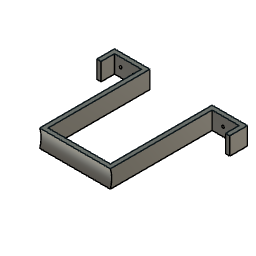
water_level_bracket_v1 (Autodesk Fusion 360 design; units mm, degrees)
Autodesk Fusion 360 part; units mm, degrees
note: some values were not read from the file. Set by a fixed rule: which sketch regions a step uses.
sketch "Sketch1" plane through (0, 0, 0) normal (0, 0, 1) x (1, 0, 0)
  line L0 (0, 0) -> (101.6, 0)
  line L1 (101.6, 0) -> (101.6, 6)
  line L2 (101.6, 6) -> (0, 6)
  line L3 (0, 6) -> (0, 0)
  dimension "d1" = 101.6
  dimension "d2" = 6
  constraint horizontal L0
  constraint vertical L1
  constraint horizontal L2
  constraint vertical L3
  constraint coincident L0.start L3.end
  measures "d1" distance of L0.start L0.end
  measures "d2" distance of L0.end L1.end
extrude "Extrude1" add sketch "Sketch1" along normal blind 25.4
sketch "Sketch2" plane through (0, 0, 25.4) normal (0, 0, 1) x (-1, 0, 0)
  line L0 (0, -6) -> (0, 0)
  line L1 (0, 0) -> (-101.6, 0)
  line L2 (-101.6, 0) -> (-101.6, -6)
  line L3 (-101.6, -6) -> (0, -6)
  line L4 (-101.6, 0) -> (-95.6, 0)
  line L5 (-95.6, 0) -> (-95.6, -152.4)
  line L6 (-95.6, -152.4) -> (-101.6, -152.4)
  line L7 (-101.6, -152.4) -> (-101.6, 0)
  dimension "d5" = 152.4
  dimension "d6" = 6
  constraint horizontal L4
  constraint vertical L5
  constraint horizontal L6
  constraint vertical L7
  constraint coincident L1.end L2.start
  measures "d5" distance of L1.end L6.end
  measures "d6" distance of L5.end L6.end
extrude "Extrude2" add sketch "Sketch2" against normal blind 25.4 contours L3 L5 L6 L7
sketch "Sketch3" plane through (0, 0, 25.4) normal (0, 0, 1) x (-1, 0, 0)
  line L0 (0, -6) -> (0, 0)
  line L1 (0, 0) -> (-101.6, 0)
  line L2 (-101.6, 0) -> (-101.6, -152.4)
  line L3 (-101.6, -152.4) -> (-95.6, -152.4)
  line L4 (-95.6, -152.4) -> (-95.6, -6)
  line L5 (-95.6, -6) -> (0, -6)
  line L6 (0, 0) -> (-6, 0)
  line L7 (-6, 0) -> (-6, -152.4)
  line L8 (-6, -152.4) -> (0, -152.4)
  line L9 (0, -152.4) -> (0, 0)
  dimension "d9" = 152.4
  dimension "d10" = 6
  constraint horizontal L6
  constraint vertical L7
  constraint horizontal L8
  constraint vertical L9
  constraint coincident L0.end L1.start
  measures "d9" distance of L0.end L8.end
  measures "d10" distance of L7.end L8.end
extrude "Extrude3" add sketch "Sketch3" against normal blind 25.4 contours L5 L7 L8 L9
sketch "Sketch4" plane through (101.6, 0, 0) normal (1, 0, 0) x (0, 1, 0)
  line L0 (0, 0) -> (152.4, 0)
  line L1 (152.4, 0) -> (152.4, 25.4)
  line L2 (152.4, 25.4) -> (0, 25.4)
  line L3 (0, 25.4) -> (0, 0)
  circle A0 centre (-39.719, 12.7) radius 41.7
  dimension "d13" = 83.4
  constraint coincident L2.end A0
  constraint coincident L0.start A0
  measures "d13" diameter of A0
extrude "Extrude4" cut sketch "Sketch4" against normal blind 101.6 contours L3 A0 picked at (0.3655, 9.8525)
sketch "Sketch5" plane through (0, 0, 25.4) normal (0, 0, 1) x (-1, 0, 0)
  line L0 (0, -152.4) -> (0, 0)
  line L1 (0, 0) -> (-101.6, 0)
  line L2 (-101.6, 0) -> (-101.6, -152.4)
  line L3 (-101.6, -152.4) -> (-95.6, -152.4)
  line L4 (-95.6, -152.4) -> (-95.6, -6)
  line L5 (-95.6, -6) -> (-6, -6)
  line L6 (-6, -6) -> (-6, -152.4)
  line L7 (-6, -152.4) -> (0, -152.4)
  line L8 (-6, -152.4) -> (44.8, -152.4)
  line L9 (44.8, -152.4) -> (44.8, -146.4)
  line L10 (44.8, -146.4) -> (-6, -146.4)
  line L11 (-6, -146.4) -> (-6, -152.4)
  dimension "d16" = 50.8
  dimension "d17" = 6
  constraint horizontal L8
  constraint vertical L9
  constraint horizontal L10
  constraint vertical L11
  constraint coincident L6.end L7.start
  measures "d16" distance of L6.end L8.end
  measures "d17" distance of L8.end L9.end
extrude "Extrude5" add sketch "Sketch5" against normal blind 25.4 contours L0 L8 L9 L10
sketch "Sketch6" plane through (0, 0, 25.4) normal (0, 0, 1) x (-1, 0, 0)
  line L0 (0, -146.4) -> (0, 0)
  line L1 (0, 0) -> (-101.6, 0)
  line L2 (-101.6, 0) -> (-101.6, -152.4)
  line L3 (-101.6, -152.4) -> (-95.6, -152.4)
  line L4 (-95.6, -152.4) -> (-95.6, -6)
  line L5 (-95.6, -6) -> (-6, -6)
  line L6 (-6, -6) -> (-6, -152.4)
  line L7 (-6, -152.4) -> (44.8, -152.4)
  line L8 (44.8, -152.4) -> (44.8, -146.4)
  line L9 (44.8, -146.4) -> (0, -146.4)
  line L10 (44.8, -152.4) -> (38.8, -152.4)
  line L11 (38.8, -152.4) -> (38.8, -127)
  line L12 (38.8, -127) -> (44.8, -127)
  line L13 (44.8, -127) -> (44.8, -152.4)
  dimension "d20" = 25.4
  dimension "d21" = 6
  constraint horizontal L10
  constraint vertical L11
  constraint horizontal L12
  constraint vertical L13
  constraint coincident L7.end L8.start
  measures "d20" distance of L7.end L12.end
  measures "d21" distance of L11.end L12.end
extrude "Extrude6" add sketch "Sketch6" against normal blind 25.4 contours L9 L11 L12 L13
sketch "Sketch7" plane through (0, 0, 25.4) normal (0, 0, 1) x (-1, 0, 0)
  line L0 (0, -146.4) -> (0, 0)
  line L1 (0, 0) -> (-101.6, 0)
  line L2 (-101.6, 0) -> (-101.6, -152.4)
  line L3 (-101.6, -152.4) -> (-95.6, -152.4)
  line L4 (-95.6, -152.4) -> (-95.6, -6)
  line L5 (-95.6, -6) -> (-6, -6)
  line L6 (-6, -6) -> (-6, -152.4)
  line L7 (-6, -152.4) -> (44.8, -152.4)
  line L8 (44.8, -152.4) -> (44.8, -127)
  line L9 (44.8, -127) -> (38.8, -127)
  line L10 (38.8, -127) -> (38.8, -146.4)
  line L11 (38.8, -146.4) -> (0, -146.4)
  line L12 (-95.6, -152.4) -> (-146.4, -152.4)
  line L13 (-146.4, -152.4) -> (-146.4, -146.4)
  line L14 (-146.4, -146.4) -> (-95.6, -146.4)
  line L15 (-95.6, -146.4) -> (-95.6, -152.4)
  dimension "d24" = 50.8
  dimension "d25" = 6
  constraint horizontal L12
  constraint vertical L13
  constraint horizontal L14
  constraint vertical L15
  constraint coincident L3.end L4.start
  measures "d24" distance of L3.end L12.end
  measures "d25" distance of L12.end L13.end
extrude "Extrude7" add sketch "Sketch7" against normal blind 25.4 contours L2 L12 L13 L14
sketch "Sketch8" plane through (0, 0, 25.4) normal (0, 0, 1) x (-1, 0, 0)
  line L0 (0, -146.4) -> (0, 0)
  line L1 (0, 0) -> (-101.6, 0)
  line L2 (-101.6, 0) -> (-101.6, -146.4)
  line L3 (-101.6, -146.4) -> (-146.4, -146.4)
  line L4 (-146.4, -146.4) -> (-146.4, -152.4)
  line L5 (-146.4, -152.4) -> (-95.6, -152.4)
  line L6 (-95.6, -152.4) -> (-95.6, -6)
  line L7 (-95.6, -6) -> (-6, -6)
  line L8 (-6, -6) -> (-6, -152.4)
  line L9 (-6, -152.4) -> (44.8, -152.4)
  line L10 (44.8, -152.4) -> (44.8, -127)
  line L11 (44.8, -127) -> (38.8, -127)
  line L12 (38.8, -127) -> (38.8, -146.4)
  line L13 (38.8, -146.4) -> (0, -146.4)
  line L14 (-146.4, -152.4) -> (-140.4, -152.4)
  line L15 (-140.4, -152.4) -> (-140.4, -127)
  line L16 (-140.4, -127) -> (-146.4, -127)
  line L17 (-146.4, -127) -> (-146.4, -152.4)
  dimension "d28" = 25.4
  dimension "d29" = 6
  constraint horizontal L14
  constraint vertical L15
  constraint horizontal L16
  constraint vertical L17
  constraint coincident L4.end L5.start
  measures "d28" distance of L4.end L16.end
  measures "d29" distance of L15.end L16.end
extrude "Extrude8" add sketch "Sketch8" against normal blind 25.4 contours L3 L15 L16 L17
sketch "Sketch9" plane through (0, 152.4, 0) normal (0, 1, 0) x (-1, 0, 0)
  line L0 (-95.6, 25.4) -> (-146.4, 25.4)
  line L1 (-146.4, 25.4) -> (-146.4, 0)
  line L2 (-146.4, 0) -> (-95.6, 0)
  line L3 (-95.6, 0) -> (-95.6, 25.4)
  circle A0 centre (-132.2412, 12.6561) radius 1.8288
  circle A1 centre (-112.7392, 12.6561) radius 1.8288
  dimension "d32" = 3.6576
  dimension "d33" = 3.6576
  measures "d32" diameter of A0
  measures "d33" diameter of A1
extrude "Extrude9" cut sketch "Sketch9" against normal blind 25 contours A0
sketch "Sketch10" plane through (0, 152.4, 0) normal (0, 1, 0) x (-1, 0, 0)
  circle A0 centre (-132.2412, 12.6561) radius 1.8288
  line L0 (-95.6, 25.4) -> (-146.4, 25.4)
  line L1 (-146.4, 25.4) -> (-146.4, 0)
  line L2 (-146.4, 0) -> (-95.6, 0)
  line L3 (-95.6, 0) -> (-95.6, 25.4)
  circle A1 centre (-117.3996, 12.4204) radius 1.8288
  dimension "d36" = 3.6576
  measures "d36" diameter of A1
extrude "Extrude10" cut sketch "Sketch10" against normal blind 30 contours A1
sketch "Sketch11" plane through (0, 152.4, 0) normal (0, 1, 0) x (-1, 0, 0)
  line L0 (44.8, 25.4) -> (-6, 25.4)
  line L1 (-6, 25.4) -> (-6, 0)
  line L2 (-6, 0) -> (44.8, 0)
  line L3 (44.8, 0) -> (44.8, 25.4)
  circle A0 centre (29.9851, 12.7) radius 1.8288
  dimension "d39" = 3.6576
  measures "d39" diameter of A0
extrude "Extrude11" cut sketch "Sketch11" against normal blind 20 contours A0
sketch "Sketch12" plane through (0, 152.4, 0) normal (0, 1, 0) x (-1, 0, 0)
  circle A0 centre (29.9851, 12.7) radius 1.8288
  line L0 (44.8, 25.4) -> (-6, 25.4)
  line L1 (-6, 25.4) -> (-6, 0)
  line L2 (-6, 0) -> (44.8, 0)
  line L3 (44.8, 0) -> (44.8, 25.4)
  circle A1 centre (10.9831, 12.9818) radius 1.8288
  dimension "d42" = 3.6576
  measures "d42" diameter of A1
extrude "Extrude12" cut sketch "Sketch12" against normal blind 30 contours A1
sketch "Sketch13" plane through (0, 0, 25.4) normal (0, 0, 1) x (-1, 0, 0)
  line L0 (0, -146.4) -> (0, 0)
  line L1 (0, 0) -> (-101.6, 0)
  line L2 (-101.6, 0) -> (-101.6, -146.4)
  line L3 (-101.6, -146.4) -> (-140.4, -146.4)
  line L4 (-140.4, -146.4) -> (-140.4, -127)
  line L5 (-140.4, -127) -> (-146.4, -127)
  line L6 (-146.4, -127) -> (-146.4, -152.4)
  line L7 (-146.4, -152.4) -> (-95.6, -152.4)
  line L8 (-95.6, -152.4) -> (-95.6, -6)
  line L9 (-95.6, -6) -> (-6, -6)
  line L10 (-6, -6) -> (-6, -152.4)
  line L11 (-6, -152.4) -> (44.8, -152.4)
  line L12 (44.8, -152.4) -> (44.8, -127)
  line L13 (44.8, -127) -> (38.8, -127)
  line L14 (38.8, -127) -> (38.8, -146.4)
  line L15 (38.8, -146.4) -> (0, -146.4)
